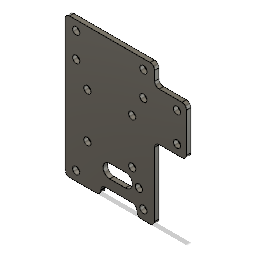
Railcore Toolchanger Layout Alpha v29 (Autodesk Fusion 360 archive; units mm, degrees)
design "Y_TC_Plate"
Autodesk Fusion 360 part; units mm, degrees
sketch "Sketch1" plane through (0, 0, 0) normal (0, 0, 1) x (1, 0, 0)
  circle A0 centre (0, 0) radius 2.5 construction
  circle A1 centre (-15, -7.25) radius 1.6
  circle A2 centre (15, -7.25) radius 1.6
  circle A3 centre (15, 35.75) radius 1.6
  circle A4 centre (-15, 35.75) radius 1.6
  circle A5 centre (10, 6.5) radius 1.6
  circle A6 centre (10, 26.5) radius 1.6
  circle A7 centre (-10, 26.5) radius 1.6
  circle A8 centre (-10, 6.5) radius 1.6
  line L0 (0, 62.6561) -> (0, -30.3688) construction
  line L1 (-27.6604, 0) -> (35.4747, 0) construction
  line L2 (-52.0325, 16.5) -> (41.5466, 16.5) construction
  circle A9 centre (-15, 46.75) radius 1.6
  circle A10 centre (15, 46.75) radius 1.6
  line L3 (-20, 51) -> (20, 51)
  line L4 (20, 51) -> (20, -11.5)
  line L5 (20, -11.5) -> (-20, -11.5)
  line L6 (-20, -11.5) -> (-20, 51)
  line L7 (-38.5408, 22.5) -> (41.7703, 22.5) construction
  circle A11 centre (30, 25.5) radius 1.6
  circle A12 centre (30, 38.5) radius 1.6
  line L8 (20, 42.75) -> (34.25, 42.75)
  line L9 (34.25, 42.75) -> (34.25, 21.25)
  line L10 (34.25, 21.25) -> (20, 21.25)
  line L11 (-4, -11.5) -> (-4, -7.25)
  line L12 (-4, -7.25) -> (12, -7.25)
  line L13 (12, -7.25) -> (12, -11.5)
  circle A13 centre (13, 0) radius 1.6
  line L14 (0, -3) -> (7, -3)
  arc A14 (7, -3) -> (7, 3) centre (7, 0) ccw
  line L15 (7, 3) -> (0, 3)
  arc A15 (0, 3) -> (0, -3) centre (0, 0) ccw
  line L16 (0, 0) -> (7, 0) construction
  dimension "d1" = 5
  dimension "d2" = 3.2
  dimension "d3" = 3.2
  dimension "d4" = 3.2
  dimension "d5" = 3.2
  dimension "d6" = 3.2
  dimension "d7" = 3.2
  dimension "d8" = 3.2
  dimension "d9" = 3.2
  dimension "d10" = 30
  dimension "d11" = 15
  dimension "d12" = 7.25
  dimension "d13" = 43
  dimension "d15" = 3.2
  dimension "d16" = 3.2
  dimension "d17" = 11
  dimension "d18" = 20
  dimension "d19" = 20
  dimension "d20" = 16.5
  dimension "d21" = 10
  dimension "d22" = 10
  dimension "d23" = 4.25
  dimension "d24" = 5
  dimension "d25" = 5
  dimension "d26" = 40
  dimension "d27" = 4.25
  dimension "d40" = 6
  dimension "d41" = 3.2
  dimension "d42" = 3.2
  dimension "d43" = 13
  dimension "d44" = 3
  dimension "d45" = 10
  dimension "d46" = 4.25
  dimension "d47" = 4.25
  dimension "d48" = 4.25
  dimension "d58" = 12
  dimension "d59" = 4
  dimension "d60" = 4.25
  dimension "d67" = 3.2
  dimension "d73" = 6
  dimension "d74" = 7
  dimension "d75" = 6
  constraint coincident A0.centre A15.centre
  constraint vertical L0
  constraint coincident A0.centre L0
  constraint perpendicular L0 L1
  constraint coincident A0.centre L1
  constraint perpendicular L0 L2
  constraint horizontal A1.centre A2.centre
  constraint vertical A1.centre A4.centre
  constraint vertical A2.centre A3.centre
  constraint horizontal A3.centre A4.centre
  constraint horizontal A9.centre A10.centre
  constraint vertical A3.centre A10.centre
  constraint vertical A4.centre A9.centre
  constraint vertical A7.centre A8.centre
  constraint vertical A5.centre A6.centre
  constraint horizontal A6.centre A7.centre
  constraint horizontal A5.centre A8.centre
  constraint horizontal L3
  constraint vertical L4
  constraint horizontal L5
  constraint vertical L6
  constraint horizontal L7
  constraint vertical A11.centre A12.centre
  constraint coincident L4 L8.start
  constraint perpendicular L4 L8
  constraint perpendicular L7 L9
  constraint coincident L4 L10.end
  constraint perpendicular L4 L10
  constraint coincident L5 L11.start
  constraint perpendicular L5 L11
  constraint perpendicular L0 L12
  constraint coincident L5 L13.end
  constraint perpendicular L5 L13
  constraint coincident L1 A13.centre
  constraint tangent L14 A14
  constraint tangent A14 L15
  constraint parallel L14 L15
  constraint tangent L15 A15
  constraint tangent L14 A15
  constraint perpendicular L0 L16
  measures "d1" diameter of A0
  measures "d2" diameter of A1
  measures "d3" diameter of A2
  measures "d4" diameter of A3
  measures "d5" diameter of A4
  measures "d6" diameter of A5
  measures "d7" diameter of A6
  measures "d8" diameter of A7
  measures "d9" diameter of A8
  measures "d10" distance of A1.centre A2.centre
  measures "d11" horizontal distance of A0.centre A1.centre
  measures "d12" vertical distance of A0.centre A2.centre
  measures "d13" distance of A2.centre A3.centre
  measures "d15" diameter of A9
  measures "d16" diameter of A10
  measures "d17" distance of A3.centre A10.centre
  measures "d18" distance of A7.centre A8.centre
  measures "d19" distance of A6.centre A7.centre
  measures "d20" vertical distance of L1.start L2.start
  measures "d21" vertical distance of A7.centre L2.start
  measures "d22" distance of A7.centre L0
  measures "d23" distance of A2.centre L5
  measures "d24" distance of A2.centre L4
  measures "d25" distance of A1.centre L6
  measures "d26" distance of L4.end L5.end
  measures "d27" distance of A9.centre L3
  measures "d40" vertical distance of L2.end L7.end
  measures "d41" diameter of A11
  measures "d42" diameter of A12
  measures "d43" distance of A11.centre A12.centre
  measures "d44" vertical distance of L7.end A11.centre
  measures "d45" distance of L4 A12.centre
  measures "d46" distance of A12.centre L8
  measures "d48" distance of A11.centre L10
  measures "d58" distance of L0 L13.end
  measures "d59" distance of L0 L11
  measures "d60" distance of L5 L12
  measures "d67" diameter of A13
  measures "d73" diameter of A14
  measures "d74" distance of A0.centre A14.centre
  measures "d75" distance of A13.centre A14.centre
extrude "Extrude1" add sketch "Sketch1" along normal blind 2 contours L3 L4 L5 L6 L11 L12 L13 | L4 L8 L9 L10
fillet "Fillet1" radius 2 8 edges at (20, 51, 1) (20, 42.75, 1) (-20, 51, 1) (34.25, 42.75, 1) (34.25, 21.25, 1) (20, 21.25, 1) (20, -11.5, 1) (-20, -11.5, 1)
fillet "Fillet1" radius 2 4 edges at (-4, -11.5, 1) (-4, -7.25, 1) (12, -7.25, 1) (12, -11.5, 1)
sketch "Sketch2" plane through (0, 0, 2) normal (0, 0, 1) x (1, 0, 0)
  arc A0 (12, -9.5) -> (14, -11.5) centre (14, -9.5) ccw
  line L0 (14, -11.5) -> (18, -11.5)
  arc A1 (18, -11.5) -> (20, -9.5) centre (18, -9.5) ccw
  line L1 (20, -9.5) -> (20, 19.25)
  arc A2 (22, 21.25) -> (20, 19.25) centre (22, 19.25) ccw
  line L2 (22, 21.25) -> (32.25, 21.25)
  arc A3 (32.25, 21.25) -> (34.25, 23.25) centre (32.25, 23.25) ccw
  line L3 (34.25, 23.25) -> (34.25, 40.75)
  arc A4 (34.25, 40.75) -> (32.25, 42.75) centre (32.25, 40.75) ccw
  line L4 (32.25, 42.75) -> (22, 42.75)
  arc A5 (20, 44.75) -> (22, 42.75) centre (22, 44.75) ccw
  line L5 (20, 44.75) -> (20, 49)
  arc A6 (20, 49) -> (18, 51) centre (18, 49) ccw
  line L6 (18, 51) -> (-18, 51)
  arc A7 (-18, 51) -> (-20, 49) centre (-18, 49) ccw
  line L7 (-20, 49) -> (-20, -9.5)
  arc A8 (-20, -9.5) -> (-18, -11.5) centre (-18, -9.5) ccw
  line L8 (-18, -11.5) -> (-6, -11.5)
  arc A9 (-6, -11.5) -> (-4, -9.5) centre (-6, -9.5) ccw
  line L9 (-4, -9.5) -> (-4, -9.25)
  arc A10 (-2, -7.25) -> (-4, -9.25) centre (-2, -9.25) ccw
  line L10 (-2, -7.25) -> (10, -7.25)
  arc A11 (12, -9.25) -> (10, -7.25) centre (10, -9.25) ccw
  line L11 (12, -9.25) -> (12, -9.5)
  circle A12 centre (30, 25.5) radius 1.6
  circle A13 centre (30, 38.5) radius 1.6
  circle A14 centre (15, 46.75) radius 1.6
  circle A15 centre (-15, 46.75) radius 1.6
  circle A16 centre (-10, 6.5) radius 1.6
  circle A17 centre (-10, 26.5) radius 1.6
  circle A18 centre (10, 26.5) radius 1.6
  circle A19 centre (10, 6.5) radius 1.6
  circle A20 centre (-15, 35.75) radius 1.6
  circle A21 centre (15, 35.75) radius 1.6
  circle A22 centre (15, -7.25) radius 1.6
  circle A23 centre (-15, -7.25) radius 1.6
  circle A24 centre (13, 0) radius 1.6
  arc A25 (0, 3) -> (0, -3) centre (0, 0) ccw
  line L12 (0, 3) -> (7, 3)
  arc A26 (7, -3) -> (7, 3) centre (7, 0) ccw
  line L13 (7, -3) -> (0, -3)
equation "d11 = d10 / 2"
equation "d21 = d18 / 2"
equation "d22 = d19 / 2"

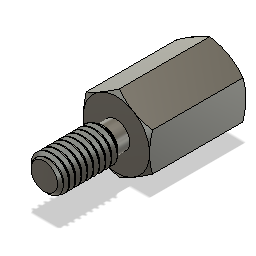
design "M3_M-F_E3D_SOFF_8L"
Autodesk Fusion 360 part; units mm, degrees
sketch "Sketch2" plane through (0, 0, 0) normal (0, 0, 1) x (1, 0, 0)
  circle A0 centre (0, 0) radius 2.75 construction
  circle A1 centre (0, 0) radius 1.05
  circle A2 centre (0, 0) radius 1.5
  line L0 (-2.75, 1.5877) -> (-2.75, -1.5877)
  line L1 (-2.75, -1.5877) -> (0, -3.1754)
  line L2 (0, -3.1754) -> (2.75, -1.5877)
  line L3 (2.75, -1.5877) -> (2.75, 1.5877)
  line L4 (2.75, 1.5877) -> (0, 3.1754)
  line L5 (0, 3.1754) -> (-2.75, 1.5877)
  dimension "d3" = 5.5
  dimension "d4" = 2.1
  dimension "d5" = 3
  dimension "d6" = 120
  dimension "d7" = 120
  constraint coincident A0.centre A1.centre
  constraint concentric A0 A1
  constraint vertical L0
  constraint parallel L0 L3
  constraint parallel L1 L4
  constraint parallel L2 L5
  constraint tangent A0 L4
  constraint tangent A0 L3
  constraint tangent A0 L5
  constraint tangent A0 L0
  constraint tangent A0 L1
  constraint tangent A0 L2
  measures "d3" diameter of A0
  measures "d4" diameter of A1
  measures "d5" diameter of A2
  measures "d6" angle of L4 L5
  measures "d7" angle of L0 L5
extrude "Extrude1" add sketch "Sketch2" along normal blind 8 contours L0 L1 L2 L3 L4 L5
extrude "Extrude4" add sketch "Sketch2" along normal blind 14 and the other way blind -6 contours A1 | A2
thread "Thread3" "ISO Metric profile 3.0 M3x0.5 6g" major diameter 2.927 minor diameter 2.3555 pitch 0.5 angle 60 modelled right hand crest width 0.0713 on face at (1.4925, -0.1494, 10) crest through (1.4635, 0, 7.875)
thread "Thread4" "ISO Metric profile 3.0 M3x0.5 6H" major diameter 3.086 minor diameter 2.529 pitch 0.5 angle 60 modelled right hand crest width 0.1368 on face at (1.4925, -0.1494, 2) crest through (1.2645, 0, 0.125)
sketch "Sketch3" plane through (0, 0, 0) normal (1, 0, 0) x (0, 0, -1)
  line L0 (-14.5, 1.1) -> (-14, 1.1)
  line L1 (-14, 1.1) -> (-13.6, 1.5)
  line L2 (-13.6, 1.5) -> (-9.4, 1.5)
  line L3 (-9.4, 1.5) -> (-9, 1.1)
  line L4 (-9, 1.1) -> (-8, 1.1)
  line L5 (-9.3255, 2.1) -> (-14.5, 2.1)
  line L6 (-14.5, 2.1) -> (-14.5, 1.1)
  line L7 (8.9461, 0) -> (-17.7087, 0) construction
  line L8 (-8, 1.1) -> (-8, 2.75)
  line L9 (-8, 2.75) -> (-7.567, 3.5)
  line L10 (-9.3255, 4.7214) -> (-9.3255, 2.1)
  line L11 (-7.567, 3.5) -> (-0.433, 3.5)
  line L12 (-0.433, 3.5) -> (0, 2.75)
  line L13 (0, 2.75) -> (0, 1.7)
  line L14 (0, 1.7) -> (-0.7345, 0.9655)
  line L15 (-0.7345, 0.9655) -> (-0.7345, 0)
  line L16 (-0.7345, 0) -> (1.568, 0)
  line L17 (1.568, 0) -> (1.568, 4.7214)
  line L18 (1.568, 4.7214) -> (-9.3255, 4.7214)
  line L19 (0, 7.4127) -> (0, -6.7444) construction
  dimension "d25" = 1.5
  dimension "d26" = 45
  dimension "d27" = 14
  dimension "d28" = 0.4
  dimension "d29" = 0.4
  dimension "d30" = 9
  dimension "d31" = 1
  dimension "d32" = 0.5
  dimension "d35" = 8
  dimension "d36" = 30
  dimension "d37" = 2.75
  dimension "d38" = 30
  dimension "d39" = 2.75
  dimension "d40" = 3.5
  dimension "d42" = 45
  dimension "d45" = 1.7
  constraint horizontal L0
  constraint parallel L0 L2
  constraint perpendicular L1 L3
  constraint parallel L2 L4
  constraint perpendicular L5 L6
  constraint horizontal L7
  constraint coincident origin L7
  constraint horizontal L5
  constraint perpendicular L4 L8
  constraint perpendicular L5 L10
  constraint horizontal L11
  constraint vertical L13
  constraint perpendicular L7 L15
  constraint perpendicular L15 L16
  constraint perpendicular L16 L17
  constraint perpendicular L10 L18
  constraint perpendicular L7 L19
  constraint coincident origin L19
  constraint coincident L12.end L19
  constraint coincident origin L16
  measures "d25" distance of L2 L7
  measures "d26" angle of L1 L2
  measures "d27" horizontal distance of origin L0.end
  measures "d28" distance of L0 L2
  measures "d29" distance of L2 L4
  measures "d30" horizontal distance of origin L3.end
  measures "d31" distance of L0.start L5.end
  measures "d32" distance of L0.start L0.end
  measures "d35" horizontal distance of origin L4.end
  measures "d36" angle of L8 L9
  measures "d37" vertical distance of origin L8.end
  measures "d38" angle of L12 L19
  measures "d39" distance of L7 L12.end
  measures "d40" distance of L7 L11
  measures "d42" angle of L13 L14
  measures "d45" distance of origin L13.end
revolve "Revolve1" cut sketch "Sketch3" angle 360 about axis through (0, 0, -8.9461) along (0, 0, 1)
equation "d29 = d28"
equation "d37 = ( 5.5 / 2 ) * 1 mm"
equation "d39 = ( 5.5 / 2 ) * 1 mm"
